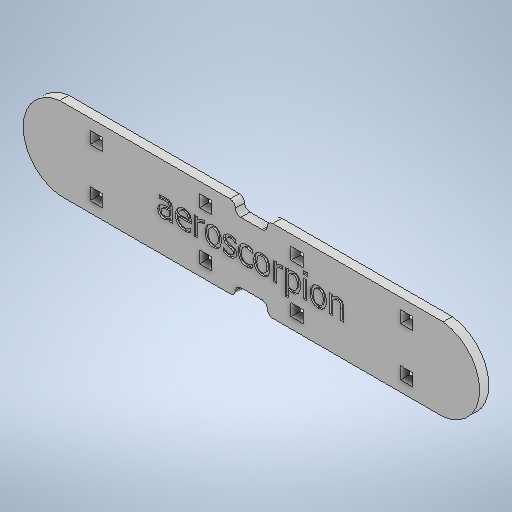
# Autodesk Inventor part: ASA_SUPERIOR
Saved by Autodesk Inventor 2025.1 (Build 291241000, 241)
## iProperties
Created: 2024-10-18
Part Number: ASA_SUPERIOR
Material: Genérico
Document SubType Name: Modeling
Designer: Aluno
Density: 1 g/cm^3
Appearance: Padrão
Author: Aluno
Autodesk Inventor part; units mm, degrees
ref_plane "YZ Plane" through (0, 0, 0) normal (1, 0, 0) x (0, 1, 0)
ref_plane "XZ Plane" through (0, 0, 0) normal (0, 1, 0) x (-1, 0, 0)
ref_plane "XY Plane" through (0, 0, 0) normal (0, 0, 1) x (1, 0, 0)
sketch "Esboço1" plane through (0, 0, 0) normal (0, 0, 1) x (1, 0, 0)
  arc A0 (-63, 13.5) -> (-75, 0) centre (-61.4062, 0) ccw
  line L0 (0, 10) -> (-3.5, 10)
  arc A1 (-5.25, 11.75) -> (-7, 13.5) centre (-7, 11.75) ccw
  arc A2 (-5.25, 11.75) -> (-3.5, 10) centre (-3.5, 11.75) ccw
  line L1 (-7, 13.5) -> (-63, 13.5)
  line L2 (-13, 10) -> (-17, 10)
  line L3 (-17, 10) -> (-17, 6)
  line L4 (-17, 6) -> (-13, 6)
  line L5 (-13, 6) -> (-13, 10)
  line L6 (-49, 10) -> (-53, 10)
  line L7 (-53, 10) -> (-53, 6)
  line L8 (-53, 6) -> (-49, 6)
  line L9 (-49, 6) -> (-49, 10)
  arc A3 (75, 0) -> (63, 13.5) centre (61.4062, 0) ccw
  line L10 (0, 10) -> (3.5, 10)
  arc A4 (7, 13.5) -> (5.25, 11.75) centre (7, 11.75) ccw
  arc A5 (3.5, 10) -> (5.25, 11.75) centre (3.5, 11.75) ccw
  line L11 (7, 13.5) -> (63, 13.5)
  line L12 (13, 10) -> (17, 10)
  line L13 (17, 10) -> (17, 6)
  line L14 (17, 6) -> (13, 6)
  line L15 (13, 6) -> (13, 10)
  line L16 (49, 10) -> (53, 10)
  line L17 (53, 10) -> (53, 6)
  line L18 (53, 6) -> (49, 6)
  line L19 (49, 6) -> (49, 10)
  arc A6 (-75, 0) -> (-63, -13.5) centre (-61.4062, 0) ccw
  line L20 (0, -10) -> (-3.5, -10)
  arc A7 (-7, -13.5) -> (-5.25, -11.75) centre (-7, -11.75) ccw
  arc A8 (-3.5, -10) -> (-5.25, -11.75) centre (-3.5, -11.75) ccw
  line L21 (-7, -13.5) -> (-63, -13.5)
  line L22 (-13, -10) -> (-17, -10)
  line L23 (-17, -10) -> (-17, -6)
  line L24 (-17, -6) -> (-13, -6)
  line L25 (-13, -6) -> (-13, -10)
  line L26 (-49, -10) -> (-53, -10)
  line L27 (-53, -10) -> (-53, -6)
  line L28 (-53, -6) -> (-49, -6)
  line L29 (-49, -6) -> (-49, -10)
  arc A9 (63, -13.5) -> (75, 0) centre (61.4062, 0) ccw
  line L30 (0, -10) -> (3.5, -10)
  arc A10 (5.25, -11.75) -> (7, -13.5) centre (7, -11.75) ccw
  arc A11 (5.25, -11.75) -> (3.5, -10) centre (3.5, -11.75) ccw
  line L31 (7, -13.5) -> (63, -13.5)
  line L32 (13, -10) -> (17, -10)
  line L33 (17, -10) -> (17, -6)
  line L34 (17, -6) -> (13, -6)
  line L35 (13, -6) -> (13, -10)
  line L36 (49, -10) -> (53, -10)
  line L37 (53, -10) -> (53, -6)
  line L38 (53, -6) -> (49, -6)
  line L39 (49, -6) -> (49, -10)
  point P0 (0, 0)
  constraints: 80 end point, 24 point on circle, 12 centre point, 4 parallel, 3 horizontal, 2 perpendicular
extrude "Extrusão1" add sketch "Esboço1" along normal blind 3
sketch "Esboço2" plane through (0, 0, 3) normal (0, 0, 1) x (1, 0, 0)
  line L0 (-32.5, 6) -> (32.5, 6) construction
  line L1 (32.5, 6) -> (32.5, -6) construction
  line L2 (32.5, -6) -> (-32.5, -6) construction
  line L3 (-32.5, -6) -> (-32.5, 6) construction
  line L4 (0, 6) -> (0, -6)
  line L5 (-32.5, 0) -> (0, 0)
  spline S0 degree 2 poles (-26.9854, -2.2853) (-27.1086, -2.376) (-27.5235, -2.7002) (-27.718, -2.7974) knots 0 0 0 1 2 2 2
  spline S1 degree 2 poles (-27.718, -2.7974) (-27.9838, -2.94) (-28.483, -3.0891) (-28.9368, -3.0891) knots 0 0 0 1 2 2 2
  spline S2 degree 2 poles (-28.9368, -3.0891) (-29.3063, -3.0891) (-29.9741, -2.8104) (-30.2269, -2.5575) knots 0 0 0 1 2 2 2
  spline S3 degree 2 poles (-30.2269, -2.5575) (-30.4668, -2.3112) (-30.7585, -1.5851) (-30.7585, -1.1831) knots 0 0 0 1 2 2 2
  spline S4 degree 2 poles (-30.7585, -1.1831) (-30.7585, -0.5608) (-30.2334, 0.3209) (-29.6629, 0.5737) knots 0 0 0 1 2 2 2
  spline S5 degree 2 poles (-29.6629, 0.5737) (-29.1572, 0.8071) (-27.7828, 0.9822) (-26.9854, 1.0276) knots 0 0 0 1 2 2 2
  line L6 (-26.9854, 1.0276) -> (-26.9854, 1.222)
  spline S6 degree 2 poles (-26.9854, 1.222) (-26.9854, 1.5721) (-27.1994, 2.0065) (-27.3938, 2.1297) knots 0 0 0 1 2 2 2
  spline S7 degree 2 poles (-27.3938, 2.1297) (-27.5883, 2.2528) (-28.1459, 2.3306) (-28.4441, 2.3306) knots 0 0 0 1 2 2 2
  spline S8 degree 2 poles (-28.4441, 2.3306) (-28.7942, 2.3306) (-29.7407, 2.1232) (-30.2139, 1.9222) knots 0 0 0 1 2 2 2
  line L7 (-30.2139, 1.9222) -> (-30.2723, 1.9222)
  line L8 (-30.2723, 1.9222) -> (-30.2723, 2.953)
  spline S9 degree 2 poles (-30.2723, 2.953) (-29.9935, 3.0308) (-28.9498, 3.2253) (-28.4376, 3.2253) knots 0 0 0 1 2 2 2
  spline S10 degree 2 poles (-28.4376, 3.2253) (-27.8152, 3.2253) (-26.966, 3.0308) (-26.6289, 2.778) knots 0 0 0 1 2 2 2
  spline S11 degree 2 poles (-26.6289, 2.778) (-26.2982, 2.5316) (-25.9741, 1.7472) (-25.9741, 1.1831) knots 0 0 0 1 2 2 2
  line L9 (-25.9741, 1.1831) -> (-25.9741, -2.9206)
  line L10 (-25.9741, -2.9206) -> (-26.9854, -2.9206)
  line L11 (-26.9854, -2.9206) -> (-26.9854, -2.2853)
  line L12 (-26.9854, -1.4425) -> (-26.9854, 0.2237)
  spline S12 degree 2 poles (-26.9854, 0.2237) (-27.3485, 0.1912) (-28.4441, 0.081) (-28.7877, -0.0227) knots 0 0 0 1 2 2 2
  spline S13 degree 2 poles (-28.7877, -0.0227) (-29.1896, -0.1459) (-29.7148, -0.658) (-29.7148, -1.1118) knots 0 0 0 1 2 2 2
  spline S14 degree 2 poles (-29.7148, -1.1118) (-29.7148, -1.6305) (-29.1313, -2.1556) (-28.5737, -2.1556) knots 0 0 0 1 2 2 2
  spline S15 degree 2 poles (-28.5737, -2.1556) (-28.1005, -2.1556) (-27.3225, -1.7472) (-26.9854, -1.4425) knots 0 0 0 1 2 2 2
  spline S16 degree 2 poles (-21.9481, -3.0567) (-23.3874, -3.0567) (-24.9692, -1.4425) (-24.9692, 0.0486) knots 0 0 0 1 2 2 2
  spline S17 degree 2 poles (-24.9692, 0.0486) (-24.9692, 1.5138) (-23.4327, 3.2512) (-22.1945, 3.2512) knots 0 0 0 1 2 2 2
  spline S18 degree 2 poles (-22.1945, 3.2512) (-21.637, 3.2512) (-20.7747, 2.9271) (-20.4571, 2.5835) knots 0 0 0 1 2 2 2
  spline S19 degree 2 poles (-20.4571, 2.5835) (-20.1329, 2.2399) (-19.7893, 1.248) (-19.7893, 0.5284) knots 0 0 0 1 2 2 2
  line L13 (-19.7893, 0.5284) -> (-19.7893, -0.0227)
  line L14 (-19.7893, -0.0227) -> (-23.9449, -0.0227)
  spline S20 degree 2 poles (-23.9449, -0.0227) (-23.9449, -1.0665) (-22.8947, -2.175) (-21.9611, -2.175) knots 0 0 0 1 2 2 2
  spline S21 degree 2 poles (-21.9611, -2.175) (-21.6305, -2.175) (-20.9887, -2.0259) (-20.7293, -1.9092) knots 0 0 0 1 2 2 2
  spline S22 degree 2 poles (-20.7293, -1.9092) (-20.4571, -1.7796) (-20.081, -1.5527) (-19.9579, -1.4489) knots 0 0 0 1 2 2 2
  line L15 (-19.9579, -1.4489) -> (-19.8995, -1.4489)
  line L16 (-19.8995, -1.4489) -> (-19.8995, -2.5511)
  spline S23 degree 2 poles (-19.8995, -2.5511) (-20.0746, -2.6224) (-20.6062, -2.8298) (-20.8136, -2.8882) knots 0 0 0 1 2 2 2
  spline S24 degree 2 poles (-20.8136, -2.8882) (-21.1054, -2.9724) (-21.5851, -3.0567) (-21.9481, -3.0567) knots 0 0 0 1 2 2 2
  spline S25 degree 2 poles (-20.7747, 0.7488) (-20.7877, 1.1572) (-20.9562, 1.7536) (-21.1183, 1.9546) knots 0 0 0 1 2 2 2
  spline S26 degree 2 poles (-21.1183, 1.9546) (-21.2934, 2.1815) (-21.8444, 2.4214) (-22.2528, 2.4214) knots 0 0 0 1 2 2 2
  spline S27 degree 2 poles (-22.2528, 2.4214) (-22.6548, 2.4214) (-23.2188, 2.1815) (-23.4522, 1.9481) knots 0 0 0 1 2 2 2
  spline S28 degree 2 poles (-23.4522, 1.9481) (-23.6791, 1.7083) (-23.9125, 1.1313) (-23.9449, 0.7488) knots 0 0 0 1 2 2 2
  line L17 (-23.9449, 0.7488) -> (-20.7747, 0.7488)
  line L18 (-15.5818, 2) -> (-15.6337, 2)
  spline S29 degree 2 poles (-15.6337, 2) (-15.7504, 2.0324) (-16.0032, 2.0454) (-16.1783, 2.0454) knots 0 0 0 1 2 2 2
  spline S30 degree 2 poles (-16.1783, 2.0454) (-16.5867, 2.0454) (-17.3906, 1.6888) (-17.7536, 1.3387) knots 0 0 0 1 2 2 2
  line L19 (-17.7536, 1.3387) -> (-17.7536, -2.9206)
  line L20 (-17.7536, -2.9206) -> (-18.765, -2.9206)
  line L21 (-18.765, -2.9206) -> (-18.765, 3.0827)
  line L22 (-18.765, 3.0827) -> (-17.7536, 3.0827)
  line L23 (-17.7536, 3.0827) -> (-17.7536, 2.188)
  spline S31 degree 2 poles (-17.7536, 2.188) (-17.2026, 2.6807) (-16.3793, 3.0827) (-15.9903, 3.0827) knots 0 0 0 1 2 2 2
  spline S32 degree 2 poles (-15.9903, 3.0827) (-15.8347, 3.0827) (-15.6791, 3.0697) (-15.5818, 3.0502) knots 0 0 0 1 2 2 2
  line L24 (-15.5818, 3.0502) -> (-15.5818, 2)
  spline S33 degree 2 poles (-9.8639, 0.081) (-9.8639, -1.436) (-11.3225, -3.0891) (-12.5413, -3.0891) knots 0 0 0 1 2 2 2
  spline S34 degree 2 poles (-12.5413, -3.0891) (-13.7925, -3.0891) (-15.2253, -1.3841) (-15.2253, 0.081) knots 0 0 0 1 2 2 2
  spline S35 degree 2 poles (-15.2253, 0.081) (-15.2253, 1.5851) (-13.7472, 3.2512) (-12.5413, 3.2512) knots 0 0 0 1 2 2 2
  spline S36 degree 2 poles (-12.5413, 3.2512) (-11.3225, 3.2512) (-9.8639, 1.5916) (-9.8639, 0.081) knots 0 0 0 1 2 2 2
  spline S37 degree 2 poles (-10.9076, 0.081) (-10.9076, 1.248) (-11.7569, 2.3825) (-12.5413, 2.3825) knots 0 0 0 1 2 2 2
  spline S38 degree 2 poles (-12.5413, 2.3825) (-13.3258, 2.3825) (-14.1815, 1.248) (-14.1815, 0.081) knots 0 0 0 1 2 2 2
  spline S39 degree 2 poles (-14.1815, 0.081) (-14.1815, -1.0535) (-13.3258, -2.2204) (-12.5413, -2.2204) knots 0 0 0 1 2 2 2
  spline S40 degree 2 poles (-12.5413, -2.2204) (-11.7634, -2.2204) (-10.9076, -1.0729) (-10.9076, 0.081) knots 0 0 0 1 2 2 2
  spline S41 degree 2 poles (-7.2058, -3.0632) (-7.8088, -3.0632) (-8.8525, -2.7391) (-9.1961, -2.5575) knots 0 0 0 1 2 2 2
  line L25 (-9.1961, -2.5575) -> (-9.1961, -1.423)
  line L26 (-9.1961, -1.423) -> (-9.1442, -1.423)
  spline S42 degree 2 poles (-9.1442, -1.423) (-9.0146, -1.5267) (-8.6645, -1.7731) (-8.3728, -1.9092) knots 0 0 0 1 2 2 2
  spline S43 degree 2 poles (-8.3728, -1.9092) (-8.1199, -2.0324) (-7.4976, -2.2139) (-7.1669, -2.2139) knots 0 0 0 1 2 2 2
  spline S44 degree 2 poles (-7.1669, -2.2139) (-6.9271, -2.2139) (-6.376, -2.1037) (-6.2464, -2.013) knots 0 0 0 1 2 2 2
  spline S45 degree 2 poles (-6.2464, -2.013) (-6.0583, -1.8898) (-5.8898, -1.611) (-5.8898, -1.3258) knots 0 0 0 1 2 2 2
  spline S46 degree 2 poles (-5.8898, -1.3258) (-5.8898, -0.9692) (-6.2788, -0.5997) (-6.778, -0.4765) knots 0 0 0 1 2 2 2
  spline S47 degree 2 poles (-6.778, -0.4765) (-6.9724, -0.4311) (-7.5948, -0.3015) (-7.8606, -0.2301) knots 0 0 0 1 2 2 2
  spline S48 degree 2 poles (-7.8606, -0.2301) (-8.5478, -0.0292) (-9.1702, 0.8006) (-9.1702, 1.3906) knots 0 0 0 1 2 2 2
  spline S49 degree 2 poles (-9.1702, 1.3906) (-9.1702, 2.2075) (-7.9449, 3.2253) (-6.9336, 3.2253) knots 0 0 0 1 2 2 2
  spline S50 degree 2 poles (-6.9336, 3.2253) (-6.4344, 3.2253) (-5.423, 2.9789) (-5.0794, 2.7909) knots 0 0 0 1 2 2 2
  line L27 (-5.0794, 2.7909) -> (-5.0794, 1.7083)
  line L28 (-5.0794, 1.7083) -> (-5.1313, 1.7083)
  spline S51 degree 2 poles (-5.1313, 1.7083) (-5.5203, 2.0194) (-6.4668, 2.376) (-6.953, 2.376) knots 0 0 0 1 2 2 2
  spline S52 degree 2 poles (-6.953, 2.376) (-7.4522, 2.376) (-8.1394, 1.9546) (-8.1394, 1.5332) knots 0 0 0 1 2 2 2
  spline S53 degree 2 poles (-8.1394, 1.5332) (-8.1394, 1.1507) (-7.731, 0.7812) (-7.2771, 0.6645) knots 0 0 0 1 2 2 2
  spline S54 degree 2 poles (-7.2771, 0.6645) (-7.0567, 0.6062) (-6.4992, 0.4895) (-6.1945, 0.4182) knots 0 0 0 1 2 2 2
  spline S55 degree 2 poles (-6.1945, 0.4182) (-5.5332, 0.2496) (-4.859, -0.5219) (-4.859, -1.1896) knots 0 0 0 1 2 2 2
  spline S56 degree 2 poles (-4.859, -1.1896) (-4.859, -1.5786) (-5.1637, -2.2658) (-5.4619, -2.5186) knots 0 0 0 1 2 2 2
  spline S57 degree 2 poles (-5.4619, -2.5186) (-5.7796, -2.7844) (-6.59, -3.0632) (-7.2058, -3.0632) knots 0 0 0 1 2 2 2
  spline S58 degree 2 poles (-1.5332, -3.0567) (-2.1556, -3.0567) (-3.1864, -2.6742) (-3.5559, -2.2853) knots 0 0 0 1 2 2 2
  spline S59 degree 2 poles (-3.5559, -2.2853) (-3.9254, -1.9028) (-4.3339, -0.7229) (-4.3339, 0.0681) knots 0 0 0 1 2 2 2
  spline S60 degree 2 poles (-4.3339, 0.0681) (-4.3339, 0.859) (-3.9125, 2.013) (-3.5559, 2.4019) knots 0 0 0 1 2 2 2
  spline S61 degree 2 poles (-3.5559, 2.4019) (-3.1994, 2.7974) (-2.1426, 3.2188) (-1.5332, 3.2188) knots 0 0 0 1 2 2 2
  spline S62 degree 2 poles (-1.5332, 3.2188) (-1.0405, 3.2188) (-0.1199, 2.94) (0.2366, 2.7585) knots 0 0 0 1 2 2 2
  line L29 (0.2366, 2.7585) -> (0.2366, 1.624)
  line L30 (0.2366, 1.624) -> (0.1783, 1.624)
  spline S63 degree 2 poles (0.1783, 1.624) (0.0681, 1.7147) (-0.269, 1.9481) (-0.5089, 2.0713) knots 0 0 0 1 2 2 2
  spline S64 degree 2 poles (-0.5089, 2.0713) (-0.7229, 2.175) (-1.2934, 2.3371) (-1.5527, 2.3371) knots 0 0 0 1 2 2 2
  spline S65 degree 2 poles (-1.5527, 2.3371) (-2.3371, 2.3371) (-3.2901, 1.1507) (-3.2901, 0.0681) knots 0 0 0 1 2 2 2
  spline S66 degree 2 poles (-3.2901, 0.0681) (-3.2901, -0.9887) (-2.3695, -2.175) (-1.5527, -2.175) knots 0 0 0 1 2 2 2
  spline S67 degree 2 poles (-1.5527, -2.175) (-1.06, -2.175) (-0.1653, -1.7666) (0.1783, -1.4489) knots 0 0 0 1 2 2 2
  line L31 (0.1783, -1.4489) -> (0.2366, -1.4489)
  line L32 (0.2366, -1.4489) -> (0.2366, -2.5835)
  spline S68 degree 2 poles (0.2366, -2.5835) (0.0875, -2.6548) (-0.3663, -2.8558) (-0.5478, -2.9011) knots 0 0 0 1 2 2 2
  spline S69 degree 2 poles (-0.5478, -2.9011) (-0.8071, -2.9789) (-1.2156, -3.0567) (-1.5332, -3.0567) knots 0 0 0 1 2 2 2
  spline S70 degree 2 poles (6.0908, 0.081) (6.0908, -1.436) (4.6321, -3.0891) (3.4133, -3.0891) knots 0 0 0 1 2 2 2
  spline S71 degree 2 poles (3.4133, -3.0891) (2.1621, -3.0891) (0.7293, -1.3841) (0.7293, 0.081) knots 0 0 0 1 2 2 2
  spline S72 degree 2 poles (0.7293, 0.081) (0.7293, 1.5851) (2.2075, 3.2512) (3.4133, 3.2512) knots 0 0 0 1 2 2 2
  spline S73 degree 2 poles (3.4133, 3.2512) (4.6321, 3.2512) (6.0908, 1.5916) (6.0908, 0.081) knots 0 0 0 1 2 2 2
  spline S74 degree 2 poles (5.047, 0.081) (5.047, 1.248) (4.1977, 2.3825) (3.4133, 2.3825) knots 0 0 0 1 2 2 2
  spline S75 degree 2 poles (3.4133, 2.3825) (2.6288, 2.3825) (1.7731, 1.248) (1.7731, 0.081) knots 0 0 0 1 2 2 2
  spline S76 degree 2 poles (1.7731, 0.081) (1.7731, -1.0535) (2.6288, -2.2204) (3.4133, -2.2204) knots 0 0 0 1 2 2 2
  spline S77 degree 2 poles (3.4133, -2.2204) (4.1912, -2.2204) (5.047, -1.0729) (5.047, 0.081) knots 0 0 0 1 2 2 2
  line L33 (10.3112, 2) -> (10.2593, 2)
  spline S78 degree 2 poles (10.2593, 2) (10.1426, 2.0324) (9.8898, 2.0454) (9.7147, 2.0454) knots 0 0 0 1 2 2 2
  spline S79 degree 2 poles (9.7147, 2.0454) (9.3063, 2.0454) (8.5024, 1.6888) (8.1394, 1.3387) knots 0 0 0 1 2 2 2
  line L34 (8.1394, 1.3387) -> (8.1394, -2.9206)
  line L35 (8.1394, -2.9206) -> (7.128, -2.9206)
  line L36 (7.128, -2.9206) -> (7.128, 3.0827)
  line L37 (7.128, 3.0827) -> (8.1394, 3.0827)
  line L38 (8.1394, 3.0827) -> (8.1394, 2.188)
  spline S80 degree 2 poles (8.1394, 2.188) (8.6904, 2.6807) (9.5138, 3.0827) (9.9028, 3.0827) knots 0 0 0 1 2 2 2
  spline S81 degree 2 poles (9.9028, 3.0827) (10.0583, 3.0827) (10.2139, 3.0697) (10.3112, 3.0502) knots 0 0 0 1 2 2 2
  line L39 (10.3112, 3.0502) -> (10.3112, 2)
  spline S82 degree 2 poles (16.1264, 0.2431) (16.1264, -1.2609) (14.6937, -3.0373) (13.5981, -3.0373) knots 0 0 0 1 2 2 2
  spline S83 degree 2 poles (13.5981, -3.0373) (13.1507, -3.0373) (12.4635, -2.8298) (12.107, -2.6159) knots 0 0 0 1 2 2 2
  line L40 (12.107, -2.6159) -> (12.107, -5.1313)
  line L41 (12.107, -5.1313) -> (11.0956, -5.1313)
  line L42 (11.0956, -5.1313) -> (11.0956, 3.0827)
  line L43 (11.0956, 3.0827) -> (12.107, 3.0827)
  line L44 (12.107, 3.0827) -> (12.107, 2.4538)
  spline S84 degree 2 poles (12.107, 2.4538) (12.483, 2.7974) (13.4036, 3.2512) (13.9417, 3.2512) knots 0 0 0 1 2 2 2
  spline S85 degree 2 poles (13.9417, 3.2512) (14.9724, 3.2512) (16.1264, 1.6175) (16.1264, 0.2431) knots 0 0 0 1 2 2 2
  spline S86 degree 2 poles (15.0827, 0.1264) (15.0827, 1.1572) (14.4279, 2.2917) (13.6953, 2.2917) knots 0 0 0 1 2 2 2
  spline S87 degree 2 poles (13.6953, 2.2917) (13.2674, 2.2917) (12.4635, 1.9092) (12.107, 1.611) knots 0 0 0 1 2 2 2
  line L45 (12.107, 1.611) -> (12.107, -1.799)
  spline S88 degree 2 poles (12.107, -1.799) (12.5024, -1.987) (13.0664, -2.1297) (13.4295, -2.1297) knots 0 0 0 1 2 2 2
  spline S89 degree 2 poles (13.4295, -2.1297) (14.2139, -2.1297) (15.0827, -0.9757) (15.0827, 0.1264) knots 0 0 0 1 2 2 2
  line L46 (18.2075, -2.9206) -> (17.1961, -2.9206)
  line L47 (17.1961, -2.9206) -> (17.1961, 3.0827)
  line L48 (17.1961, 3.0827) -> (18.2075, 3.0827)
  line L49 (18.2075, 3.0827) -> (18.2075, -2.9206)
  line L50 (18.2788, 4.081) -> (17.1313, 4.081)
  line L51 (17.1313, 4.081) -> (17.1313, 5.1313)
  line L52 (17.1313, 5.1313) -> (18.2788, 5.1313)
  line L53 (18.2788, 5.1313) -> (18.2788, 4.081)
  spline S90 degree 2 poles (24.6256, 0.081) (24.6256, -1.436) (23.1669, -3.0891) (21.9481, -3.0891) knots 0 0 0 1 2 2 2
  spline S91 degree 2 poles (21.9481, -3.0891) (20.6969, -3.0891) (19.2642, -1.3841) (19.2642, 0.081) knots 0 0 0 1 2 2 2
  spline S92 degree 2 poles (19.2642, 0.081) (19.2642, 1.5851) (20.7423, 3.2512) (21.9481, 3.2512) knots 0 0 0 1 2 2 2
  spline S93 degree 2 poles (21.9481, 3.2512) (23.1669, 3.2512) (24.6256, 1.5916) (24.6256, 0.081) knots 0 0 0 1 2 2 2
  spline S94 degree 2 poles (23.5818, 0.081) (23.5818, 1.248) (22.7326, 2.3825) (21.9481, 2.3825) knots 0 0 0 1 2 2 2
  spline S95 degree 2 poles (21.9481, 2.3825) (21.1637, 2.3825) (20.3079, 1.248) (20.3079, 0.081) knots 0 0 0 1 2 2 2
  spline S96 degree 2 poles (20.3079, 0.081) (20.3079, -1.0535) (21.1637, -2.2204) (21.9481, -2.2204) knots 0 0 0 1 2 2 2
  spline S97 degree 2 poles (21.9481, -2.2204) (22.7261, -2.2204) (23.5818, -1.0729) (23.5818, 0.081) knots 0 0 0 1 2 2 2
  line L54 (30.376, -2.9206) -> (29.3647, -2.9206)
  line L55 (29.3647, -2.9206) -> (29.3647, 0.5024)
  spline S98 degree 2 poles (29.3647, 0.5024) (29.3647, 0.9173) (29.2869, 1.6305) (29.1702, 1.8444) knots 0 0 0 1 2 2 2
  spline S99 degree 2 poles (29.1702, 1.8444) (29.047, 2.0713) (28.6062, 2.2917) (28.2301, 2.2917) knots 0 0 0 1 2 2 2
  spline S100 degree 2 poles (28.2301, 2.2917) (27.8541, 2.2917) (27.0567, 1.8898) (26.6742, 1.5656) knots 0 0 0 1 2 2 2
  line L56 (26.6742, 1.5656) -> (26.6742, -2.9206)
  line L57 (26.6742, -2.9206) -> (25.6629, -2.9206)
  line L58 (25.6629, -2.9206) -> (25.6629, 3.0827)
  line L59 (25.6629, 3.0827) -> (26.6742, 3.0827)
  line L60 (26.6742, 3.0827) -> (26.6742, 2.4149)
  spline S101 degree 2 poles (26.6742, 2.4149) (27.128, 2.8233) (28.0032, 3.2512) (28.4959, 3.2512) knots 0 0 0 1 2 2 2
  spline S102 degree 2 poles (28.4959, 3.2512) (29.3776, 3.2512) (30.376, 2.0843) (30.376, 0.9757) knots 0 0 0 1 2 2 2
  line L61 (30.376, 0.9757) -> (30.376, -2.9206)
  point P0 (0, 0)
  point P1 (32.5, 0)
  dimension "d23" = 65
  dimension "d24" = 12
  constraints: 5 midpoint, 4 end point, 1 vertical, 2 other
  measures "d23" distance of point (32.5, 0) L5.start
  measures "d24" distance of L4.end L4.start
extrude "Extrusão2" cut sketch "Esboço2" against normal blind 0.5 contours S62 L29 L30 S63 L4 | L4 S63 S64 S65 S66 L5 S59 S60 S61 S62 | S67 L31 L32 S68 L4 | L4 S68 S69 S58 S59 L5 S66 S67 | S4 S5 L6 S6 S7 S8 L7 L8 S9 S10 S11 L9 L5 L12 S12 | L5 S12 S13 S14 S15 L12 L9 L10 L11 S0 S1 S2 S3 S4 | S16 S17 S18 S19 L13 L5 | L5 L13 L14 S20 S21 S22 L15 L16 S23 S24 S16 | L21 L22 L23 S31 S32 L24 L18 S29 S30 L19 L5 | L5 L19 L20 L21 | S34 S35 S36 S33 L5 S40 S37 S38 S39 | L5 S39 S40 S33 S34 | S48 S49 S50 L27 L28 S51 S52 S53 S54 S55 L5 | L5 S55 S56 S57 S41 L25 L26 S42 S43 S44 S45 S46 S47 S48 | S70 S71 S72 S73 | L33 S78 S79 L34 L35 L36 L37 L38 S80 S81 L39 | S82 S83 L40 L41 L42 L43 L44 S84 S85 | L46 L47 L48 L49 | L50 L51 L52 L53 | S90 S91 S92 S93 | L54 L55 S98 S99 S100 L56 L57 L58 L59 L60 S101 S102 L61
